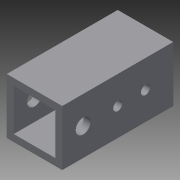
# Autodesk Inventor part: Clapper Inner Cable Hard Stop (2)
Saved by Autodesk Inventor 2014 (Build 180170000, 170)
## iProperties
Created: 2014-02-24
Part Number: Clapper Inner Cable Hard Stop (2)
Material: Generic
Document SubType Name: Modeling
Designer: Michael
Density: 1 g/cm^3
Appearance: Default
Author: Michael
Autodesk Inventor part; units mm, degrees
ref_plane "YZ Plane" through (0, 0, 0) normal (1, 0, 0) x (0, 1, 0)
ref_plane "XZ Plane" through (0, 0, 0) normal (0, 1, 0) x (-1, 0, 0)
ref_plane "XY Plane" through (0, 0, 0) normal (0, 0, 1) x (1, 0, 0)
sketch "Sketch1" plane through (0, 0, 0) normal (0, 0, 1) x (1, 0, 0)
  line L0 (0, 0) -> (25.4, 0)
  line L1 (25.4, 0) -> (25.4, 25.4)
  line L2 (25.4, 25.4) -> (0, 25.4)
  line L3 (0, 25.4) -> (0, 0)
  line L4 (22.225, 3.175) -> (3.175, 3.175)
  line L5 (3.175, 3.175) -> (3.175, 22.225)
  line L6 (3.175, 22.225) -> (22.225, 22.225)
  line L7 (22.225, 22.225) -> (22.225, 3.175)
  dimension "d0" = 25.4
  dimension "d1" = 25.4
  dimension "d2" = 3.175
  constraints: 16 end point, 4 parallel, 2 perpendicular, 1 horizontal, 3 other
  measures "d0" distance of L2.end L1.end
  measures "d1" distance of L1.end L0.end
  measures "d2" distance between parallel lines of L0 L4
extrude "Extrusion1" add sketch "Sketch1" along normal blind 50.8
sketch "Sketch2" plane through (25.4, 0, 0) normal (1, 0, 0) x (0, 0, -1)
  line L0 (0, 0) -> (0, 25.4) projected
  line L1 (-50.8, 0) -> (-50.8, 25.4) projected
  line L2 (0, 0) -> (-50.8, 0) projected
  circle A0 centre (-41.275, 12.7) radius 3.3782
  circle A1 centre (-12.7, 12.7) radius 2.0701
  circle A2 centre (-25.4, 12.7) radius 2.0701
  dimension "d5" = 6.7564
  dimension "d6" = 12.7
  dimension "d7" = 9.525
  dimension "d8" = 4.1402
  dimension "d9" = 12.7
  dimension "d10" = 12.7
  dimension "d13" = 12.7
  constraints: 3 centre point, 1 horizontal, 2 other
  measures "d5" diameter of A0
  measures "d6" distance from line of L2 A0.centre
  measures "d7" distance from line of L1 A0.centre
  measures "d8" diameter of A1
  measures "d9" distance from line of L0 A1.centre
  measures "d10" distance from line of L2 A1.centre
  measures "d13" distance of A1.centre A2.centre
extrude "Extrusion2" cut sketch "Sketch2" against normal blind 50.8
body "Solid1"
